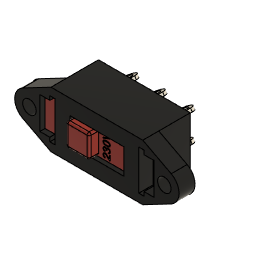
T22205B436B (Autodesk Fusion 360 design; units mm, degrees)
Autodesk Fusion 360 part; units mm, degrees
sketch "Skizze1" plane through (0, 0, 0) normal (0, 1, 0) x (1, 0, 0)
  line L0 (11.5, 7) -> (-11.5, 7)
  line L1 (-11.5, 7) -> (-11.5, -7)
  line L2 (-11.5, -7) -> (11.5, -7)
  line L3 (11.5, -7) -> (11.5, 7)
  line L4 (11.5, 7) -> (-11.5, -7) construction
  line L5 (-11.5, 7) -> (11.5, -7) construction
  line L6 (6.75, 3.2) -> (-6.75, 3.2)
  line L7 (-6.75, 3.2) -> (-6.75, -3.2)
  line L8 (-6.75, -3.2) -> (6.75, -3.2)
  line L9 (6.75, -3.2) -> (6.75, 3.2)
  line L10 (6.75, 3.2) -> (-6.75, -3.2) construction
  line L11 (-6.75, 3.2) -> (6.75, -3.2) construction
  line L12 (-5.95, 2.9) -> (-1.15, 2.9)
  line L13 (-0.65, 2.4) -> (-0.65, -2.4)
  line L14 (-1.15, -2.9) -> (-5.95, -2.9)
  line L15 (-6.45, -2.4) -> (-6.45, 2.4)
  line L16 (0, 0) -> (-16.3534, 0) construction
  circle A0 centre (-16.9, 0) radius 1.7
  circle A1 centre (16.9, 0) radius 1.7
  line L17 (0, 0) -> (0, -6.4356) construction
  line L18 (-11.5, -7) -> (-18.6149, -3.2786)
  line L19 (-11.5, 7) -> (-18.6149, 3.2786)
  line L20 (11.5, -7) -> (18.6149, -3.2786)
  line L21 (11.5, 7) -> (18.6149, 3.2786)
  arc A2 (-1.15, -2.9) -> (-0.65, -2.4) centre (-1.15, -2.4) ccw
  arc A3 (-0.65, 2.4) -> (-1.15, 2.9) centre (-1.15, 2.4) ccw
  arc A4 (-6.45, -2.4) -> (-5.95, -2.9) centre (-5.95, -2.4) ccw
  arc A5 (-5.95, 2.9) -> (-6.45, 2.4) centre (-5.95, 2.4) ccw
  line L22 (10.5, -5) -> (10.5, 5)
  arc A6 (18.6149, -3.2786) -> (18.6149, 3.2786) centre (16.9, 0) ccw
  arc A7 (-18.6149, 3.2786) -> (-18.6149, -3.2786) centre (-16.9, 0) ccw
  line L23 (14.3, -4) -> (14.3, 4)
  line L24 (10.5, -5) -> (11.8, -5)
  line L25 (10.5, 5) -> (11.8, 5)
  line L26 (14.3, -4) -> (11.8, -4)
  line L27 (11.8, -4) -> (11.8, -5)
  line L28 (14.3, 4) -> (11.8, 4)
  line L29 (11.8, 4) -> (11.8, 5)
  line L30 (-10.5, -5) -> (-10.5, 5)
  line L31 (-10.5, 5) -> (-11.8, 5)
  line L32 (-11.8, 5) -> (-11.8, 4)
  line L33 (-11.8, 4) -> (-14.3, 4)
  line L34 (-14.3, 4) -> (-14.3, -4)
  line L35 (-14.3, -4) -> (-11.8, -4)
  line L36 (-11.8, -4) -> (-11.8, -5)
  line L37 (-11.8, -5) -> (-10.5, -5)
  line L38 (2.2845, 2.7624) -> (2.2845, -2.9834) construction
  line L39 (2.2845, -2.9834) -> (-0.2155, -2.9834) construction
  line L40 (-0.2155, -2.9834) -> (-0.2155, 2.7624) construction
  line L41 (-0.2155, 2.7624) -> (2.2845, 2.7624) construction
  point P0 (-6.45, 2.9)
  point P1 (-0.65, 2.9)
  point P2 (-6.45, -2.9)
  point P3 (17.255, 0)
  dimension "d1" = 23
  dimension "d2" = 14
  dimension "d3" = 13.5
  dimension "d4" = 6.4
  dimension "d5" = 5.8
  dimension "d6" = 5.8
  dimension "d7" = 0.3
  dimension "d8" = 3.4
  dimension "d9" = 16.9
  dimension "d10" = 7.4
  dimension "d12" = 33.8
  dimension "d20" = 0.5
  dimension "d21" = 0.5
  dimension "d22" = 0.5
  dimension "d23" = 0.5
  dimension "d27" = 10
  dimension "d28" = 10.5
  dimension "d29" = 3.7
  dimension "d30" = 8
  dimension "d31" = 3.8
  dimension "d32" = 1.3
  dimension "d33" = 1.3
  text T0 "230V" font "Arial" height 2.5 align ink ink in box 0 x 0 at (2.2845, 2.7624) x (0, -1) y (-1, 0) spacing 1 kerned height is em
  constraint perpendicular L0 L1
  constraint parallel L0 L2
  constraint parallel L1 L3
  constraint horizontal L0
  constraint coincident L4 L16.start
  constraint coincident L5 L16.start
  constraint coincident L16.start L17.start
  constraint perpendicular L6 L7
  constraint parallel L6 L8
  constraint parallel L7 L9
  constraint horizontal L6
  constraint coincident L10 L16.start
  constraint coincident L11 L16.start
  constraint horizontal L12
  constraint vertical L13
  constraint horizontal L14
  constraint vertical L15
  constraint perpendicular L1 L16
  constraint symmetric L12 L14 L16
  constraint perpendicular L2 L17
  constraint symmetric A0 A1 L17
  constraint concentric A0 A7
  constraint concentric A1 A6
  constraint tangent L18 A7
  constraint tangent L19 A7
  constraint tangent L20 A6
  constraint tangent L21 A6
  constraint tangent L13 A2
  constraint tangent L14 A2
  constraint coincident P1 L12
  constraint coincident P1 L13
  constraint tangent L12 A3
  constraint tangent L13 A3
  constraint coincident P2 L14
  constraint coincident P2 L15
  constraint tangent L14 A4
  constraint tangent L15 A4
  constraint coincident P0 L12
  constraint coincident P0 L15
  constraint tangent L12 A5
  constraint tangent L15 A5
  constraint parallel L9 L22
  constraint symmetric L16 L22.start L22.end
  constraint parallel L3 L23
  constraint symmetric L16 L23.start L23.end
  constraint perpendicular L3 L24
  constraint perpendicular L3 L25
  constraint perpendicular L3 L26
  constraint perpendicular L24 L27
  constraint perpendicular L23 L28
  constraint perpendicular L25 L29
  constraint perpendicular L16 L30
  constraint perpendicular L1 L31
  constraint perpendicular L16 L32
  constraint perpendicular L1 L33
  constraint perpendicular L16 L34
  constraint perpendicular L34 L35
  constraint perpendicular L16 L36
  constraint symmetric L17 L22 L30
  constraint symmetric L17 L23 L34
  constraint symmetric L17 L24 L37
  constraint symmetric L17 L25 L31
  constraint symmetric L17 L26 L35
  constraint symmetric L17 L28 L33
  constraint symmetric L17 L27 L36
  constraint symmetric L17 L29 L32
  constraint perpendicular L38 L39
  constraint parallel L38 L40
  constraint parallel L39 L41
  measures "d1" distance of L1.end L2.end
  measures "d2" distance of L0.end L1.end
  measures "d3" distance of L7.end L8.end
  measures "d4" distance of L6.end L7.end
  measures "d5" distance of P0 P1
  measures "d6" distance of P0 P2
  measures "d7" distance of L7 L15
  measures "d8" diameter of A0
  measures "d9" distance of L16.start A0.centre
  measures "d10" diameter of A7
  measures "d12" distance of A0.centre A1.centre
  measures "d20" radius of A2
  measures "d21" radius of A3
  measures "d22" radius of A4
  measures "d23" radius of A5
  measures "d27" distance of L22.start L22.end
  measures "d28" distance of L16.start L22
  measures "d29" radius of A6
  measures "d30" distance of L23.start L23.end
  measures "d31" distance of L22 L23
  measures "d32" distance of L22.start L24.end
  measures "d33" distance of L22.end L25.end
extrude "Extrusion1" add sketch "Skizze1" along normal blind 4 contours L3 L20 L21 A6 L23 L24 L25 L26 L27 L28 L29 | L1 L18 L19 A7 L31 L32 L33 L34 L35 L36 L37 | L3 L23 L24 L25 L26 L27 L28 L29 | L1 L31 L32 L33 L34 L35 L36 L37 makes body 1 at (-12.7333, 0, 0) makes body 2 at (12.7333, 0, 0)
extrude "Extrusion2" add sketch "Skizze1" along normal blind 11.9 contours L0 L1 L2 L3 L22 L24 L25 L30 L31 L37 | L3 L22 L24 L25 | L1 L30 L31 L37 | L6 L7 L8 L9 | L12 L13 L14 L15 A2 A3 A4 A5 bodies 1 2
extrude "Extrusion3" cut sketch "Skizze1" along normal blind 1.1 contours L6 L7 L8 L9 bodies 1
extrude "Extrusion4" add sketch "Skizze1" against normal blind 1.3 contours L12 L13 L14 L15 A2 A3 A4 A5 bodies 1
fillet "Abrundung1" radius 0.5 8 edges at (-0.65, -1.3, 0) (-0.7964, -1.3, 2.7536) (-3.55, -1.3, 2.9) (-6.3036, -1.3, 2.7536) (-6.45, -1.3, 0) (-6.3036, -1.3, -2.7536) (-3.55, -1.3, -2.9) (-0.7964, -1.3, -2.7536) on bodies 1
extrude "Extrusion5" cut sketch "Skizze1" along normal blind 1.3 contours L1 L30 L31 L37 | L1 L31 L32 L33 L34 L35 L36 L37 bodies 1
extrude "Extrusion6" cut sketch "Skizze1" along normal blind 3.6 contours L3 L23 L24 L25 L26 L27 L28 L29 | L3 L22 L24 L25 bodies 1
sketch "Skizze2" plane through (0, 11.9, 0) normal (0, 1, 0) x (-1, 0, 0)
  line L0 (-11.5, 7) -> (-11.5, -7)
  line L1 (-11.5, -7) -> (11.5, -7)
  line L2 (11.5, -7) -> (11.5, 7)
  line L3 (11.5, 7) -> (-11.5, 7)
  line L4 (10.9, -6.3) -> (-10.9, -6.3)
  line L5 (-10.9, -6.3) -> (-10.9, 6.3)
  line L6 (-10.9, 6.3) -> (10.9, 6.3)
  line L7 (10.9, 6.3) -> (10.9, -6.3)
  line L8 (10.9, -6.3) -> (-10.9, 6.3) construction
  line L9 (-10.9, -6.3) -> (10.9, 6.3) construction
  line L10 (0, 0) -> (0, 12.3227) construction
  line L11 (0, 0) -> (13.0204, 0) construction
  line L12 (1.5, 3.9) -> (-1.5, 3.9)
  line L13 (-1.5, 3.9) -> (-1.5, 3.1)
  line L14 (-1.5, 3.1) -> (1.5, 3.1)
  line L15 (1.5, 3.1) -> (1.5, 3.9)
  line L16 (1.5, 3.9) -> (-1.5, 3.1) construction
  line L17 (-1.5, 3.9) -> (1.5, 3.1) construction
  line L18 (1.5, -3.1) -> (-1.5, -3.1)
  line L19 (-1.5, -3.1) -> (-1.5, -3.9)
  line L20 (-1.5, -3.9) -> (1.5, -3.9)
  line L21 (1.5, -3.9) -> (1.5, -3.1)
  line L22 (1.5, -3.1) -> (-1.5, -3.9) construction
  line L23 (-1.5, -3.1) -> (1.5, -3.9) construction
  line L24 (-5.5, 3.1) -> (-8.5, 3.1)
  line L25 (-8.5, 3.1) -> (-8.5, 3.9)
  line L26 (-8.5, 3.9) -> (-5.5, 3.9)
  line L27 (-5.5, 3.9) -> (-5.5, 3.1)
  line L28 (-5.5, 3.1) -> (-8.5, 3.9) construction
  line L29 (-8.5, 3.1) -> (-5.5, 3.9) construction
  line L30 (8.5, 3.1) -> (5.5, 3.1)
  line L31 (5.5, 3.1) -> (5.5, 3.9)
  line L32 (5.5, 3.9) -> (8.5, 3.9)
  line L33 (8.5, 3.9) -> (8.5, 3.1)
  line L34 (8.5, 3.1) -> (5.5, 3.9) construction
  line L35 (5.5, 3.1) -> (8.5, 3.9) construction
  line L36 (-5.5, -3.9) -> (-8.5, -3.9)
  line L37 (-8.5, -3.9) -> (-8.5, -3.1)
  line L38 (-8.5, -3.1) -> (-5.5, -3.1)
  line L39 (-5.5, -3.1) -> (-5.5, -3.9)
  line L40 (-5.5, -3.9) -> (-8.5, -3.1) construction
  line L41 (-8.5, -3.9) -> (-5.5, -3.1) construction
  line L42 (8.5, -3.1) -> (5.5, -3.1)
  line L43 (5.5, -3.1) -> (5.5, -3.9)
  line L44 (5.5, -3.9) -> (8.5, -3.9)
  line L45 (8.5, -3.9) -> (8.5, -3.1)
  line L46 (8.5, -3.1) -> (5.5, -3.9) construction
  line L47 (5.5, -3.1) -> (8.5, -3.9) construction
  point P0 (0, 3.5)
  point P1 (0, -3.5)
  point P2 (-7, 3.5)
  point P3 (7, 3.5)
  point P4 (-7, -3.5)
  point P5 (7, -3.5)
  dimension "d38" = 12.6
  dimension "d39" = 21.8
  dimension "d42" = 3
  dimension "d43" = 0.8
  dimension "d44" = 3.5
  dimension "d45" = 7
  dimension "d46" = 3
  dimension "d47" = 3
  dimension "d48" = 7
  constraint perpendicular L4 L5
  constraint parallel L4 L6
  constraint parallel L5 L7
  constraint horizontal L4
  constraint coincident L8 L10.start
  constraint coincident L9 L10.start
  constraint coincident L10.start L11.start
  constraint perpendicular L3 L10
  constraint perpendicular L2 L11
  constraint perpendicular L12 L13
  constraint parallel L12 L14
  constraint parallel L13 L15
  constraint horizontal L12
  constraint coincident L16 P0
  constraint coincident L17 P0
  constraint coincident L10 P0
  constraint perpendicular L18 L19
  constraint parallel L18 L20
  constraint parallel L19 L21
  constraint horizontal L18
  constraint coincident L22 P1
  constraint coincident L23 P1
  constraint symmetric L11 P0 P1
  constraint symmetric L11 L12 L20
  constraint symmetric L11 L15 L21
  constraint perpendicular L24 L25
  constraint parallel L24 L26
  constraint parallel L25 L27
  constraint horizontal L24
  constraint coincident L28 P2
  constraint coincident L29 P2
  constraint collinear L12 L26
  constraint collinear L14 L24
  constraint perpendicular L30 L31
  constraint parallel L30 L32
  constraint parallel L31 L33
  constraint horizontal L30
  constraint coincident L34 P3
  constraint coincident L35 P3
  constraint collinear L12 L32
  constraint collinear L14 L30
  constraint perpendicular L36 L37
  constraint parallel L36 L38
  constraint parallel L37 L39
  constraint horizontal L36
  constraint coincident L40 P4
  constraint coincident L41 P4
  constraint collinear L27 L39
  constraint collinear L25 L37
  constraint collinear L20 L36
  constraint collinear L18 L38
  constraint perpendicular L42 L43
  constraint parallel L42 L44
  constraint parallel L43 L45
  constraint horizontal L42
  constraint coincident L46 P5
  constraint coincident L47 P5
  constraint collinear L31 L43
  constraint collinear L33 L45
  constraint collinear L18 L42
  constraint collinear L20 L44
  measures "d38" distance of L4.end L5.end
  measures "d39" distance of L5 L7
  measures "d42" distance of L13.end L14.end
  measures "d43" distance of L12.end L13.end
  measures "d44" distance of L10.start P0
  measures "d45" distance of P0 P2
  measures "d46" distance of L25.end L26.end
  measures "d47" distance of L31 L33
  measures "d48" distance of P0 P3
extrude "Extrusion7" cut sketch "Skizze2" against normal blind 1.3 contours L4 L5 L6 L7 bodies 1
extrude "Extrusion8" add 1 faces at (-0.5, 11.9, -3.6333) along direction (0, 1, 0) blind 5 separate body on bodies 1 makes body 3
fillet "Abrundung2" radius 1.5 2 edges at (-1.5, 16.9, -3.5) (1.5, 16.9, -3.5) on bodies 3
sketch "Skizze3" plane through (0, 0, -3.1) normal (0, 0, 1) x (-1, 0, 0)
  arc A0 (-1.5, -15.4) -> (1.5, -15.4) centre (0, -15.4) ccw
  line L0 (1.5, -15.4) -> (1.5, -11.9)
  line L1 (1.5, -11.9) -> (-1.5, -11.9)
  line L2 (-1.5, -11.9) -> (-1.5, -15.4)
  line L3 (0, -15.4) -> (0, -11.4313) construction
  line L4 (0.7, -15.4) -> (0.7, -14.2)
  line L5 (-0.7, -15.4) -> (-0.7, -14.2)
  arc A1 (-0.7, -15.4) -> (0.7, -15.4) centre (0, -15.4) ccw
  arc A2 (0.7, -14.2) -> (-0.7, -14.2) centre (0, -14.2) ccw
  line L6 (11.5, -11.9) -> (-11.5, -11.9)
  arc A3 (1.5, -12.35) -> (1.5, -13.65) centre (1.5, -13) ccw
  arc A4 (-1.5, -13.65) -> (-1.5, -12.35) centre (-1.5, -13) ccw
  dimension "d55" = 0.8
  dimension "d56" = 1.2
  dimension "d60" = 1.1
  dimension "d62" = 0.65
  constraint coincident A0.centre L3.start
  constraint perpendicular L1 L3
  constraint concentric A0 A1
  constraint coincident L3 A2.centre
  constraint equal A1 A2
  constraint tangent L4 A2
  constraint parallel L3 L4
  constraint tangent L5 A2
  constraint parallel L2 L5
  constraint coincident L2 A4.centre
  constraint coincident L0 A3.centre
  constraint symmetric L3 A3 A4
  constraint coincident L0 A3.end
  constraint coincident L0 A3.start
  constraint coincident L2 A4.end
  constraint coincident L2 A4.start
  measures "d55" distance of A0 A1
  measures "d56" distance of A0.centre A2.centre
  measures "d60" distance of A4.centre L6
  measures "d62" radius of A4
extrude "Extrusion9" cut sketch "Skizze3" against normal blind 0.8 contours A0 L0 L1 L2 L6 A3 A4 | L2 A4 | L0 A3 | L4 L5 A1 A2 bodies 3
extrude "Extrusion10" add sketch "Skizze3" against normal blind 0.8 separate body contours A0 L0 L1 L2 L6 A3 A4 makes body 4
extrude "Extrusion11" cut 6 faces at (-7.5, 11.9, -3.6333) (-0.5, 11.9, -3.6333) (6.5, 11.9, -3.6333) (7.5, 11.9, 3.3667) (-0.5, 11.9, 3.3667) (-7.5, 11.9, 3.3667) along direction (0, -1, 0) blind 1.5 on bodies 1 bodies 1
extrude "Extrusion12" add 1 faces at (-0.5, 11.9, -3.3667) along direction (0, -1, 0) blind 1.3 on bodies 4 bodies 4 3
move_body "Verschieben6" bodies 4 to x (1, 0, 0) y (0, 1, 0) z (0, 0, 1) at (0, 0, 3.5)
move_body "Verschieben7" bodies 4 to x (0.866025, 0, 0.5) y (0, 1, 0) z (-0.5, 0, 0.866025) at (-0.401, 0, 0.6964)
move_body "Verschieben8" bodies 4 to x (1, 0, 0) y (0, 1, 0) z (0, 0, 1) at (-0.0392, 0, -2.6622)
move_body "Verschieben9" bodies 4 to x (1, 0, 0) y (0, 1, 0) z (0, 0, 1) at (0.0318, -0.0087, -0.0344)
move_body "Verschieben13" bodies 4 to x (1, 0, 0) y (0, 1, 0) z (0, 0, 1) at (0.4, 0, -1.5)
copy_body "Körper kopieren/einfügen6" bodies 4 makes body 5
move_body "Verschieben10" bodies 5 to x (1, 0, 0) y (0, 1, 0) z (0, 0, 1) at (0, 0, 7)
copy_body "Körper kopieren/einfügen7" bodies 4 5 makes body 6 makes body 7
move_body "Verschieben11" bodies 6 7 to x (1, 0, 0) y (0, 1, 0) z (0, 0, 1) at (7, 0, 0)
copy_body "Körper kopieren/einfügen8" bodies 4 5 makes body 8 makes body 9
move_body "Verschieben12" bodies 8 9 to x (1, 0, 0) y (0, 1, 0) z (0, 0, 1) at (-7, 0, 0)
combine "Kombinieren1" operation add target body 1 tool bodies 4 5 6 7 8 9
copy_body "Körper kopieren/einfügen2" bodies 1 makes body 10
copy_body "Körper kopieren/einfügen3" bodies 1 makes body 11
combine "Kombinieren2" operation add target body 1 tool bodies 10 11
extrude "Extrusion13" cut sketch "Skizze1" along normal blind 1.35 text T0 bodies 1
copy_body "Körper kopieren/einfügen4" [suppressed]
copy_body "Körper kopieren/einfügen5" [suppressed]
equation "d29 = d10 / 2"
equation "d33 = d32"
equation "d46 = d42"
equation "d47 = d42"
equation "d48 = d45"
named bodies: "switch", "solder latch", "solder latch (1) (1)", "solder latch (1) (1) (1)", "solder latch (1) (2)", "solder latch (1)", "solder latch (3)", "solder latch (1) (3)", "solder latch (4)", "solder latch (1) (4)", "switch (1)", "switch (1) (1)"
